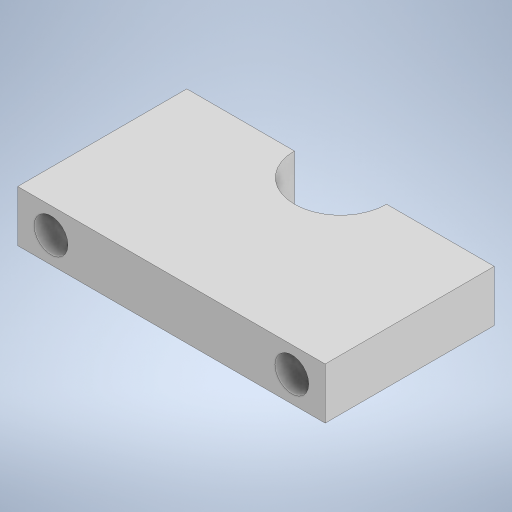
# Autodesk Inventor part: Steher oben Rohr
Saved by Autodesk Inventor 2024 (Build 280153000, 153)
## iProperties
Created: 2024-03-08
Part Number: Steher oben Rohr
Material: Generisch
Document SubType Name: Modeling
Designer: Andreas Weber
Density: 1 g/cm^3
Appearance: Vorgabe
Author: Andreas Weber
Autodesk Inventor part; units mm, degrees
ref_plane "YZ Plane" through (0, 0, 0) normal (1, 0, 0) x (0, 1, 0)
ref_plane "XZ Plane" through (0, 0, 0) normal (0, 1, 0) x (-1, 0, 0)
sketch "Skizze1" plane through (0, 0, 0) normal (0, 0, 1) x (1, 0, 0)
  line L0 (0, 0) -> (60, 0)
  line L1 (60, 0) -> (60, -150)
  line L2 (60, -150) -> (0, -150)
  line L3 (0, -150) -> (0, 0)
  circle A0 centre (30, -117) radius 9
  dimension "d0" = 60
  dimension "d1" = 150
  dimension "d2" = 18
  constraints: 8 end point, 2 parallel, 1 centre point, 1 coincident, 1 horizontal, 1 perpendicular
  measures "d0" distance of L1.end L2.end
  measures "d1" distance of L0.end L1.end
  measures "d2" diameter of A0
extrude "Extrusion1" add sketch "Skizze1" along normal blind 10
sketch "Skizze2" plane through (0, -150, 0) normal (0, -1, 0) x (1, 0, 0)
  point P0 (0, 0)
  point P1 (6.5, 5)
  point P2 (53.5, 5)
sketch "Skizze3" plane through (0, 0, 0) normal (0, 0, -1) x (-1, 0, 0)
  line L0 (-5, -117) -> (-55, -117)
  point P0 (0, 0)
  constraints: 2 end point, 1 horizontal
ref_plane "Arbeitsebene1" through (5, -117, 0) normal (0, 1, 0) x (1, 0, 0)
split "Trennen1" plane through (5, -117, 0) removes the side toward (0, 1, 0)
hole "Bohrung2" at (6.5, -150, 5) at (53.5, -150, 5) direction (0, 1, 0) diameter 6.6 end through all
